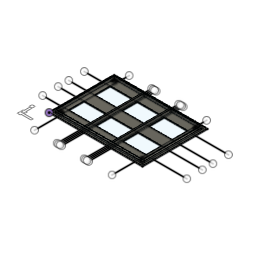
Freedeck_Lid_V1.1 (Autodesk Fusion 360 design; units mm, degrees)
Autodesk Fusion 360 part; units mm, degrees
sketch "Sketch1" plane through (0, 0, 0) normal (0, 0, 1) x (1, 0, 0)
  line L0 (0, 0) -> (103.6, 0)
  line L1 (103.6, 0) -> (103.6, 72.2)
  line L2 (103.6, 72.2) -> (0, 72.2)
  line L3 (0, 72.2) -> (0, 0)
  line L4 (94.8, 80) -> (94.8, -25)
  line L5 (68.8, 80) -> (68.8, -25)
  line L6 (63.8, 80) -> (63.8, -25)
  line L7 (38.8, 80) -> (38.8, -25)
  line L8 (33.8, 80) -> (33.8, -25)
  line L9 (8.8, 80) -> (8.8, -25)
  line L10 (-20, 59) -> (140, 59)
  line L11 (-20, 41.8) -> (140, 41.8)
  line L12 (-20, 30) -> (140, 30)
  line L13 (-20, 12.8) -> (140, 12.8)
  line L14 (2.5, 69.7) -> (101.15, 69.7)
  line L15 (101.15, 69.7) -> (101.15, 2.45)
  line L16 (101.15, 2.45) -> (2.5, 2.45)
  line L17 (2.5, 2.45) -> (2.5, 69.7)
  line L18 (4.1, 68.1) -> (99.55, 68.1)
  line L19 (99.55, 68.1) -> (99.55, 4.05)
  line L20 (99.55, 4.05) -> (4.1, 4.05)
  line L21 (4.1, 4.05) -> (4.1, 68.1)
  line L22 (35.5, 80) -> (35.5, -25)
  line L23 (37.1, -25) -> (37.1, 80)
  line L24 (65.5, 80) -> (65.5, -25)
  line L25 (67.1, -25) -> (67.1, 80)
  circle A0 centre (6.5, 65.9) radius 1.6
  circle A1 centre (97.3, 65.8) radius 1.6
  circle A2 centre (97.2, 6.1) radius 1.6
  circle A3 centre (6.5, 6.3) radius 1.6
  dimension "d1" = 103.6
  dimension "d2" = 72.2
  dimension "d3" = 8.8
  dimension "d4" = 26
  dimension "d5" = 5
  dimension "d7" = 5
  dimension "d8" = 25
  dimension "d10" = 8.8
  dimension "d11" = 25
  dimension "d12" = 17.2
  dimension "d13" = 17.2
  dimension "d14" = 11.8
  dimension "d15" = 12.8
  dimension "d16" = 13.2
  dimension "d17" = 2.5
  dimension "d18" = 2.5
  dimension "d19" = 2.45
  dimension "d20" = 2.45
  dimension "d21" = 1.6
  dimension "d22" = 1.6
  dimension "d23" = 1.6
  dimension "d24" = 1.6
  dimension "d37" = 1.6
  dimension "d38" = 1.7
  dimension "d39" = 1.7
  dimension "d40" = 1.6
  dimension "d41" = 1.7
  dimension "d44" = 3.2
  dimension "d45" = 6.5
  dimension "d46" = 6.3
  dimension "d47" = 3.2
  dimension "d48" = 6.3
  dimension "d49" = 6.4
  dimension "d50" = 3.2
  dimension "d51" = 6.4
  dimension "d52" = 6.1
  dimension "d53" = 3.2
  dimension "d54" = 6.5
  dimension "d55" = 6.3
  constraint horizontal L0
  constraint vertical L1
  constraint horizontal L2
  constraint vertical L3
  constraint coincident L0.start L3.end
  constraint perpendicular L2 L4
  constraint horizontal L11
  constraint horizontal L12
  constraint perpendicular L1 L13
  constraint horizontal L14
  constraint vertical L15
  constraint horizontal L16
  constraint vertical L17
  constraint horizontal L18
  constraint vertical L19
  constraint horizontal L20
  constraint vertical L21
  constraint perpendicular L16 L22
  constraint parallel L7 L23
  measures "d1" distance of L0.start L0.end
  measures "d2" distance of L0.end L1.end
  measures "d3" distance of L1 L4
  measures "d4" distance of L4 L5
  measures "d5" distance of L5 L6
  measures "d7" distance of L7 L8
  measures "d8" distance of L8 L9
  measures "d10" distance of L3 L9
  measures "d11" distance of L6 L7
  measures "d12" distance of L10 L11
  measures "d13" distance of L12 L13
  measures "d14" distance of L11 L12
  measures "d15" distance of L0 L13
  measures "d16" distance of L2 L10
  measures "d17" distance of L2 L14
  measures "d18" distance of L3 L17
  measures "d19" distance of L0 L16
  measures "d20" distance of L1 L15
  measures "d21" distance of L17 L21
  measures "d22" distance of L14 L18
  measures "d23" distance of L15 L19
  measures "d24" distance of L16 L20
  measures "d37" distance of L22 L23
  measures "d38" distance of L7 L23
  measures "d39" distance of L8 L22
  measures "d40" distance of L24 L25
  measures "d41" distance of L6 L24
  measures "d44" diameter of A0
  measures "d45" distance of L3 A0.centre
  measures "d46" distance of L2 A0.centre
  measures "d47" diameter of A1
  measures "d48" distance of L1 A1.centre
  measures "d49" distance of L2 A1.centre
  measures "d50" diameter of A2
  measures "d51" distance of L1 A2.centre
  measures "d52" distance of L0 A2.centre
  measures "d53" diameter of A3
  measures "d54" distance of L3 A3.centre
  measures "d55" distance of L0 A3.centre
extrude "Extrude1" add sketch "Sketch1" along normal blind 0.64 contours L0 L3 L9 L13 L16 L17 | L0 L8 L9 L16 | L3 L12 L13 L17 | L0 L8 L16 L22 | L9 L13 L16 L17 L20 L21 | L8 L9 L16 L20 | L3 L11 L12 L17 | L12 L13 L17 L21 | L0 L16 L22 L23 | L8 L16 L20 L22 | L9 L13 L20 L21 | L8 L9 L13 L20 | L3 L10 L11 L17 | L11 L12 L17 L21 | L9 L12 L13 L21 | L0 L7 L16 L23 | L16 L20 L22 L23 | L8 L13 L20 L22 | L2 L3 L9 L10 L14 L17 | L10 L11 L17 L21 | L9 L11 L12 L21 | L0 L6 L7 L16 | L7 L16 L20 L23 | L13 L20 L22 L23 | L8 L12 L13 L22 | L8 L9 L11 L12 | L9 L10 L14 L17 L18 L21 | L9 L10 L11 L21 | L0 L6 L16 L24 | L6 L7 L16 L20 | L7 L13 L20 L23 | L12 L13 L22 L23 | L8 L11 L12 L22 | L2 L8 L9 L14 | L9 L10 L18 L21 | L0 L16 L24 L25 | L6 L16 L20 L24 | L6 L7 L13 L20 | L7 L12 L13 L23 | L11 L12 L22 L23 | L8 L10 L11 L22 | L8 L9 L10 L18 | L2 L8 L14 L22 | L8 L9 L14 L18 | L0 L5 L16 L25 | L16 L20 L24 L25 | L6 L13 L20 L24 | L7 L11 L12 L23 | L10 L11 L22 L23 | L8 L10 L18 L22 | L2 L14 L22 L23 | L8 L14 L18 L22 | L0 L4 L5 L16 | L5 L16 L20 L25 | L13 L20 L24 L25 | L6 L12 L13 L24 | L6 L7 L11 L12 | L7 L10 L11 L23 | L10 L18 L22 L23 | L2 L7 L14 L23 | L14 L18 L22 L23 | L0 L1 L4 L13 L15 L16 | L4 L5 L16 L20 | L5 L13 L20 L25 | L12 L13 L24 L25 | L6 L11 L12 L24 | L7 L10 L18 L23 | L2 L6 L7 L14 | L7 L14 L18 L23 | L4 L13 L15 L16 L19 L20 | L4 L5 L13 L20 | L5 L12 L13 L25 | L11 L12 L24 L25 | L6 L10 L11 L24 | L6 L7 L10 L18 | L2 L6 L14 L24 | L6 L7 L14 L18 | L1 L12 L13 L15 | L4 L13 L19 L20 | L5 L11 L12 L25 | L10 L11 L24 L25 | L6 L10 L18 L24 | L2 L14 L24 L25 | L6 L14 L18 L24 | L1 L11 L12 L15 | L12 L13 L15 L19 | L4 L12 L13 L19 | L4 L5 L11 L12 | L5 L10 L11 L25 | L10 L18 L24 L25 | L2 L5 L14 L25 | L14 L18 L24 L25 | L1 L10 L11 L15 | L11 L12 L15 L19 | L4 L11 L12 L19 | L5 L10 L18 L25 | L2 L4 L5 L14 | L5 L14 L18 L25 | L1 L2 L4 L10 L14 L15 | L10 L11 L15 L19 | L4 L10 L11 L19 | L4 L5 L10 L18 | L4 L5 L14 L18 | L4 L10 L14 L15 L18 L19 | L4 L10 L18 L19 | A0 | A1 | A2 | A3 makes body 1
extrude "Extrude2" add sketch "Sketch1" along normal blind 3 separate body contours L9 L13 L16 L17 L20 L21 | L8 L9 L16 L20 | L12 L13 L17 L21 | L8 L16 L20 L22 | L11 L12 L17 L21 | L16 L20 L22 L23 | L10 L11 L17 L21 | L7 L16 L20 L23 | L9 L10 L14 L17 L18 L21 | L6 L7 L16 L20 | L6 L16 L20 L24 | L8 L9 L14 L18 | L16 L20 L24 L25 | L8 L14 L18 L22 | L5 L16 L20 L25 | L14 L18 L22 L23 | L4 L5 L16 L20 | L7 L14 L18 L23 | L4 L13 L15 L16 L19 L20 | L6 L7 L14 L18 | L6 L14 L18 L24 | L12 L13 L15 L19 | L14 L18 L24 L25 | L11 L12 L15 L19 | L5 L14 L18 L25 | L10 L11 L15 L19 | L4 L5 L14 L18 | L4 L10 L14 L15 L18 L19 makes body 2
fillet "Fillet1" radius 3 4 edges at (103.6, 0, 0.32) (103.6, 72.2, 0.32) (0, 0, 0.32) (0, 72.2, 0.32) on bodies 1 2
fillet "Fillet1" radius 2 4 edges at (2.5, 69.7, 1.5) (2.5, 2.45, 1.5) (101.15, 2.45, 1.5) (101.15, 69.7, 1.5) on bodies 1 2
fillet "Fillet2" radius 0.5 8 edges at (51.8, 72.2, 0) (0.8787, 71.3213, 0) (0, 36.1, 0) (0.8787, 0.8787, 0) (51.8, 0, 0) (102.7213, 0.8787, 0) (103.6, 36.1, 0) (102.7213, 71.3213, 0) on bodies 1
fillet "Fillet3" radius 1 8 edges at (100.5642, 69.1142, 3) (51.825, 69.7, 3) (3.0858, 69.1142, 3) (2.5, 36.075, 3) (3.0858, 3.0358, 3) (51.825, 2.45, 3) (100.5642, 3.0358, 3) (101.15, 36.075, 3) on bodies 2
extrude "Extrude3" add sketch "Sketch1" along normal blind 3 separate body contours L13 L20 L22 L23 | L12 L13 L22 L23 | L11 L12 L22 L23 | L10 L11 L22 L23 | L13 L20 L24 L25 | L10 L18 L22 L23 | L12 L13 L24 L25 | L11 L12 L24 L25 | L10 L11 L24 L25 | L10 L18 L24 L25 makes body 3 at (35.5, 46.75, 1) makes body 4 at (65.5, 46.75, 1)
equation "d10 = d3"
equation "d12 = d13"
equation "d18 = d17"
